Autodesk Fusion 360 part; units mm, degrees
(part 5 of 8)
  spline S792 degree 3 poles (24.0351, 9.5293) (23.3482, 9.5293) (23.0556, 8.9736) (22.8466, 8.9736) knots 0 0 0 0 1 1 1 1
  spline S793 degree 3 poles (22.8466, 8.9736) (22.2105, 8.9736) (21.3624, 9.9262) (21.3624, 10.7728) knots 0 0 0 0 1 1 1 1
  spline S794 degree 3 poles (21.3624, 10.7728) (21.3624, 11.8842) (22.739, 13.0748) (24.3546, 13.0748) knots 0 0 0 0 1 1 1 1
  spline S795 degree 3 poles (24.3546, 13.0748) (26.2837, 13.0748) (27.8455, 11.3814) (27.8455, 9.3176) knots 0 0 0 0 1 1 1 1
  spline S796 degree 3 poles (27.8455, 9.3176) (27.8455, 7.413) (26.8204, 6.2798) (25.0116, 5.8403) knots 0 0 0 0 0.899792 0.899792 0.899792 0.899792
  spline S797 degree 3 poles (25.0116, 5.8403) (24.8102, 5.7914) (24.5991, 5.751) (24.3785, 5.7192) knots 0.899792 0.899792 0.899792 0.899792 1 1 1 1
  spline S798 degree 3 poles (24.3785, 5.7192) (25.0522, 5.3732) (25.6655, 4.9493) (26.2098, 4.4555) knots 0 0 0 0 0.233548 0.233548 0.233548 0.233548
  ellipse E21 centre (19.5885, -1.7408) end of major axis (19.5885, -11.5568) minor radius 8.5372 (19.5885, -11.5568) -> (26.2098, 4.4555) ccw
  spline S799 degree 3 poles (19.5885, -11.5568) (19.4017, -11.5543) (19.2169, -11.5473) (19.0342, -11.5361) knots 0.009853 0.009853 0.009853 0.009853 0.044162 0.044162 0.044162 0.044162
  spline S800 degree 3 poles (207.0718, -10.6848) (207.0718, -10.1028) (207.4951, -6.9807) (207.4951, -6.769) knots 0 0 0 0 1 1 1 1
  spline S801 degree 3 poles (207.4951, -6.769) (207.4951, -6.9807) (207.0718, -10.1028) (207.0718, -10.6848) knots -1 -1 -1 -1 0 0 0 0
  spline S802 degree 3 poles (9.0107, -11.2935) (7.9525, -11.2406) (6.6827, -11.2142) (5.5155, -11.2142) knots 0 0 0 0 1 1 1 1
  spline S803 degree 3 poles (5.5155, -11.2142) (6.6827, -11.2142) (7.9525, -11.2406) (9.0107, -11.2935) knots -1 -1 -1 -1 0 0 0 0
  spline S804 degree 3 poles (-20.2282, 3.0734) (-20.1993, 0.0308) (-10.7804, 0.4806) (-10.7804, -6.1341) knots 0 0 0 0 1 1 1 1
  spline S805 degree 3 poles (-10.7804, -6.1341) (-10.7804, 0.4806) (-20.1993, 0.0308) (-20.2282, 3.0734) knots -1 -1 -1 -1 0 0 0 0
  spline S806 degree 3 poles (25.2803, 8.4181) (25.2803, 9.0001) (24.9608, 9.5293) (24.0351, 9.5293) knots 0 0 0 0 1 1 1 1
  spline S807 degree 3 poles (24.0351, 9.5293) (24.9608, 9.5293) (25.2803, 9.0001) (25.2803, 8.4181) knots -1 -1 -1 -1 0 0 0 0
  spline S808 degree 3 poles (312.7442, 4.1318) (313.1411, 5.2166) (311.4213, 5.1902) (311.4213, 5.587) knots 0 0 0 0 1 1 1 1
  spline S809 degree 3 poles (311.4213, 5.587) (311.4213, 5.1902) (313.1411, 5.2166) (312.7442, 4.1318) knots -1 -1 -1 -1 0 0 0 0
  spline S810 degree 3 poles (-61.1571, -0.6308) (-61.1571, 4.158) (-58.5644, 6.7775) (-53.9628, 6.7775) knots 0 0 0 0 0.999995 0.999995 0.999995 0.999995
  spline S811 degree 3 poles (-53.9628, 6.7775) (-58.5644, 6.7775) (-61.1571, 4.158) (-61.1571, -0.6308) knots -0.999995 -0.999995 -0.999995 -0.999995 0 0 0 0
  line L198 (311.1567, -0.3132) -> (306.2614, -0.2867)
  line L199 (306.2614, -0.2867) -> (308.7223, -7.2188)
  line L200 (308.7223, -7.2188) -> (311.1567, -0.3132)
  line L201 (305.6267, 1.5654) -> (311.8446, 1.6183)
  line L202 (311.8446, 1.6183) -> (312.7442, 4.1318)
  spline S812 degree 3 poles (312.7442, 4.1318) (313.1411, 5.2166) (311.4213, 5.1902) (311.4213, 5.587) knots 0 0 0 0 1 1 1 1
  spline S813 degree 3 poles (311.4213, 5.587) (311.4213, 5.9045) (311.7123, 6.5131) (311.924, 6.4866) knots 0 0 0 0 1 1 1 1
  spline S814 degree 3 poles (311.924, 6.4866) (312.3209, 6.4337) (313.1149, 6.4072) (313.9086, 6.4072) knots 0 0 0 0 1 1 1 1
  spline S815 degree 3 poles (313.9086, 6.4072) (314.7024, 6.4072) (315.4961, 6.4337) (315.893, 6.4866) knots 0 0 0 0 1 1 1 1
  spline S816 degree 3 poles (315.893, 6.4866) (316.1311, 6.5131) (316.3957, 5.9045) (316.3957, 5.587) knots 0 0 0 0 1 1 1 1
  spline S817 degree 3 poles (316.3957, 5.587) (316.3957, 5.1902) (315.2051, 5.1902) (314.8347, 4.1318) knots 0 0 0 0 1 1 1 1
  line L203 (314.8347, 4.1318) -> (309.9129, -9.6794)
  spline S818 degree 3 poles (309.9129, -9.6794) (310.3627, -10.0234) (310.8919, -10.1557) (310.8919, -10.4203) knots 0 0 0 0 1 1 1 1
  spline S819 degree 3 poles (310.8919, -10.4203) (310.8919, -10.7378) (310.6011, -11.3225) (310.3894, -11.2934) knots 0 0 0 0 1 1 1 1
  spline S820 degree 3 poles (310.3894, -11.2934) (308.5106, -11.1346) (306.4998, -11.2934) (305.5999, -11.2934) knots 0 0 0 0 1 1 1 1
  spline S821 degree 3 poles (305.5999, -11.2934) (304.7003, -11.2934) (304.4358, -11.1346) (304.277, -10.6848) knots 0 0 0 0 1 1 1 1
  line L204 (304.277, -10.6848) -> (299.0115, 4.1318)
  spline S822 degree 3 poles (299.0115, 4.1318) (298.6411, 5.2166) (297.4505, 5.1902) (297.4505, 5.587) knots 0 0 0 0 1 1 1 1
  spline S823 degree 3 poles (297.4505, 5.587) (297.4505, 5.9045) (297.7151, 6.4866) (297.9265, 6.4866) knots 0 0 0 0 1 1 1 1
  spline S824 degree 3 poles (297.9265, 6.4866) (298.9851, 6.4337) (300.3609, 6.4072) (301.737, 6.4072) knots 0 0 0 0 1 1 1 1
  spline S825 degree 3 poles (301.737, 6.4072) (303.1129, 6.4072) (304.4622, 6.4337) (305.5206, 6.4866) knots 0 0 0 0 1 1 1 1
  spline S826 degree 3 poles (305.5206, 6.4866) (305.7322, 6.4866) (306.0235, 5.9045) (306.0235, 5.587) knots 0 0 0 0 1 1 1 1
  spline S827 degree 3 poles (306.0235, 5.587) (306.0235, 5.1902) (304.3299, 5.2166) (304.7004, 4.1318) knots 0 0 0 0 1 1 1 1
  line L205 (304.7004, 4.1318) -> (305.6267, 1.5654)
  line L206 (-32.4486, -8.7797) -> (-32.4486, 4.1582)
  line L207 (-32.4486, 4.1582) -> (-32.4486, -8.7797)
  spline S828 degree 3 poles (27.8455, 9.3176) (27.8455, 7.413) (26.8204, 6.2798) (25.0116, 5.8403) knots 0 0 0 0 0.899792 0.899792 0.899792 0.899792
  spline S829 degree 3 poles (25.0116, 5.8403) (26.8204, 6.2798) (27.8455, 7.413) (27.8455, 9.3176) knots -0.899792 -0.899792 -0.899792 -0.899792 0 0 0 0
  line L208 (182.2539, -3.885) -> (182.2539, -8.965)
  line L209 (182.2539, -8.965) -> (182.2539, -3.885)
  spline S830 degree 3 poles (180.7986, -10.4203) (180.7986, -10.0234) (182.2539, -10.1028) (182.2539, -8.965) knots 0 0 0 0 1 1 1 1
  line L210 (182.2539, -8.965) -> (182.2539, -3.885)
  line L211 (182.2539, -3.885) -> (175.9039, -3.885)
  line L212 (175.9039, -3.885) -> (175.9039, -8.965)
  spline S831 degree 3 poles (175.9039, -8.965) (175.9039, -10.0763) (177.3326, -9.9969) (177.3326, -10.4203) knots 0 0 0 0 1 1 1 1
  spline S832 degree 3 poles (177.3326, -10.4203) (177.3326, -10.7378) (177.068, -11.3225) (176.8564, -11.2934) knots 0 0 0 0 1 1 1 1
  spline S833 degree 3 poles (176.8564, -11.2934) (175.798, -11.2405) (174.5016, -11.214) (173.2316, -11.214) knots 0 0 0 0 1 1 1 1
  spline S834 degree 3 poles (173.2316, -11.214) (171.9351, -11.214) (170.6386, -11.2405) (169.6068, -11.2934) knots 0 0 0 0 1 1 1 1
  spline S835 degree 3 poles (169.6068, -11.2934) (169.3951, -11.3225) (169.1041, -10.7378) (169.1041, -10.4203) knots 0 0 0 0 1 1 1 1
  spline S836 degree 3 poles (169.1041, -10.4203) (169.1041, -9.9969) (170.5593, -10.0763) (170.5593, -8.965) knots 0 0 0 0 1 1 1 1
  line L213 (170.5593, -8.965) -> (170.5593, 4.1583)
  spline S837 degree 3 poles (170.5593, 4.1583) (170.5593, 5.296) (169.1041, 5.2166) (169.1041, 5.64) knots 0 0 0 0 1 1 1 1
  spline S838 degree 3 poles (169.1041, 5.64) (169.1041, 5.9575) (169.3951, 6.5131) (169.6068, 6.5131) knots 0 0 0 0 1 1 1 1
  spline S839 degree 3 poles (169.6068, 6.5131) (170.6386, 6.4602) (171.9351, 6.4337) (173.2316, 6.4337) knots 0 0 0 0 1 1 1 1
  spline S840 degree 3 poles (173.2316, 6.4337) (174.5016, 6.4337) (175.798, 6.4602) (176.8564, 6.5131) knots 0 0 0 0 1 1 1 1
  spline S841 degree 3 poles (176.8564, 6.5131) (177.068, 6.5131) (177.3326, 5.9575) (177.3326, 5.64) knots 0 0 0 0 1 1 1 1
  spline S842 degree 3 poles (177.3326, 5.64) (177.3326, 5.2166) (175.9039, 5.296) (175.9039, 4.1583) knots 0 0 0 0 1 1 1 1
  line L214 (175.9039, 4.1583) -> (175.9039, -1.9007)
  line L215 (175.9039, -1.9007) -> (182.2539, -1.9007)
  line L216 (182.2539, -1.9007) -> (182.2539, 4.1583)
  spline S843 degree 3 poles (182.2539, 4.1583) (182.2539, 5.296) (180.7986, 5.2166) (180.7986, 5.64) knots 0 0 0 0 1 1 1 1
  spline S844 degree 3 poles (180.7986, 5.64) (180.7986, 5.9575) (181.0897, 6.5131) (181.3014, 6.5131) knots 0 0 0 0 1 1 1 1
  spline S845 degree 3 poles (181.3014, 6.5131) (182.3332, 6.4602) (183.6297, 6.4337) (184.8997, 6.4337) knots 0 0 0 0 1 1 1 1
  spline S846 degree 3 poles (184.8997, 6.4337) (186.1961, 6.4337) (187.4661, 6.4602) (188.5245, 6.5131) knots 0 0 0 0 1 1 1 1
  spline S847 degree 3 poles (188.5245, 6.5131) (188.7626, 6.5131) (189.0272, 5.9575) (189.0272, 5.64) knots 0 0 0 0 1 1 1 1
  spline S848 degree 3 poles (189.0272, 5.64) (189.0272, 5.2166) (187.5984, 5.296) (187.5984, 4.1583) knots 0 0 0 0 1 1 1 1
  line L217 (187.5984, 4.1583) -> (187.5984, -8.965)
  spline S849 degree 3 poles (187.5984, -8.965) (187.5984, -10.0763) (189.0272, -9.9969) (189.0272, -10.4203) knots 0 0 0 0 1 1 1 1
  spline S850 degree 3 poles (189.0272, -10.4203) (189.0272, -10.7378) (188.7626, -11.3225) (188.5245, -11.2934) knots 0 0 0 0 1 1 1 1
  spline S851 degree 3 poles (188.5245, -11.2934) (187.4661, -11.2405) (186.1961, -11.214) (184.8997, -11.214) knots 0 0 0 0 1 1 1 1
  spline S852 degree 3 poles (184.8997, -11.214) (183.6297, -11.214) (182.3332, -11.2405) (181.3014, -11.2934) knots 0 0 0 0 1 1 1 1
  spline S853 degree 3 poles (181.3014, -11.2934) (181.0897, -11.3225) (180.7986, -10.7378) (180.7986, -10.4203) knots 0 0 0 0 1 1 1 1
  spline S854 degree 3 poles (-62.1118, -11.2935) (-62.3212, -11.3227) (-62.5342, -10.7379) (-62.5342, -10.4202) knots 0 0 0 0 1 1 1 1
  spline S855 degree 3 poles (-62.5342, -10.4202) (-62.5342, -10.7379) (-62.3212, -11.3227) (-62.1118, -11.2935) knots -1 -1 -1 -1 0 0 0 0
  spline S856 degree 3 poles (-8.269, 4.1319) (-8.851, 5.1107) (-10.096, 5.2165) (-10.096, 5.6134) knots 0 0 0 0 1 1 1 1
  spline S857 degree 3 poles (-10.096, 5.6134) (-10.096, 5.2165) (-8.851, 5.1107) (-8.269, 4.1319) knots -1 -1 -1 -1 0 0 0 0
  spline S858 degree 3 poles (25.0116, 5.8403) (24.8102, 5.7914) (24.5991, 5.751) (24.3785, 5.7192) knots 0.899792 0.899792 0.899792 0.899792 1 1 1 1
  spline S859 degree 3 poles (24.3785, 5.7192) (24.5991, 5.751) (24.8102, 5.7914) (25.0116, 5.8403) knots -1 -1 -1 -1 -0.899792 -0.899792 -0.899792 -0.899792
  spline S860 degree 3 poles (112.6975, 5.6135) (112.6975, 5.2166) (111.5334, 5.296) (111.3746, 4.1583) knots 0 0 0 0 1 1 1 1
  spline S861 degree 3 poles (111.3746, 4.1583) (111.5334, 5.296) (112.6975, 5.2166) (112.6975, 5.6135) knots -1 -1 -1 -1 0 0 0 0
  spline S862 degree 3 poles (208.3682, -6.2663) (208.8709, -6.2663) (208.9503, -9.3619) (213.7393, -9.3619) knots 0 0 0 0 1 1 1 1
  spline S863 degree 3 poles (213.7393, -9.3619) (208.9503, -9.3619) (208.8709, -6.2663) (208.3682, -6.2663) knots -1 -1 -1 -1 0 0 0 0
  spline S864 degree 3 poles (16.2828, -2.3771) (16.2828, 2.518) (17.3668, 4.9254) (19.7498, 4.9254) knots -1 -1 -1 -1 0 0 0 0
  spline S865 degree 3 poles (19.7498, 4.9254) (22.1298, 4.9254) (23.2168, 2.518) (23.2168, -2.3771) knots -1 -1 -1 -1 0 0 0 0
  spline S866 degree 3 poles (23.2168, -2.3771) (23.2168, -7.2718) (22.1298, -9.7058) (19.7498, -9.7058) knots -1 -1 -1 -1 0 0 0 0
  spline S867 degree 3 poles (19.7498, -9.7058) (17.3937, -9.7058) (16.2828, -7.3512) (16.2828, -2.3771) knots -1 -1 -1 -1 0 0 0 0
  ellipse E22 centre (19.5885, -1.7408) end of major axis (19.5885, -11.5568) minor radius 8.5372 (12.3354, 3.4367) -> (19.0342, -11.5361) ccw
  spline S868 degree 3 poles (19.0342, -11.5361) (19.2169, -11.5473) (19.4017, -11.5543) (19.5885, -11.5568) knots -0.044162 -0.044162 -0.044162 -0.044162 -0.009853 -0.009853 -0.009853 -0.009853
  ellipse E23 centre (19.5885, -1.7408) end of major axis (19.5885, -11.5568) minor radius 8.5372 (19.5885, -11.5568) -> (26.2098, 4.4555) ccw
  spline S869 degree 3 poles (26.2098, 4.4555) (25.6655, 4.9493) (25.0522, 5.3732) (24.3785, 5.7192) knots -0.233548 -0.233548 -0.233548 -0.233548 0 0 0 0
  spline S870 degree 3 poles (24.3785, 5.7192) (24.5991, 5.751) (24.8102, 5.7914) (25.0116, 5.8403) knots -1 -1 -1 -1 -0.899792 -0.899792 -0.899792 -0.899792
  spline S871 degree 3 poles (25.0116, 5.8403) (26.8204, 6.2798) (27.8455, 7.413) (27.8455, 9.3176) knots -0.899792 -0.899792 -0.899792 -0.899792 0 0 0 0
  spline S872 degree 3 poles (27.8455, 9.3176) (27.8455, 11.3814) (26.2837, 13.0748) (24.3546, 13.0748) knots -1 -1 -1 -1 0 0 0 0
  spline S873 degree 3 poles (24.3546, 13.0748) (22.739, 13.0748) (21.3624, 11.8842) (21.3624, 10.7728) knots -1 -1 -1 -1 0 0 0 0
  spline S874 degree 3 poles (21.3624, 10.7728) (21.3624, 9.9262) (22.2105, 8.9736) (22.8466, 8.9736) knots -1 -1 -1 -1 0 0 0 0
  spline S875 degree 3 poles (22.8466, 8.9736) (23.0556, 8.9736) (23.3482, 9.5293) (24.0351, 9.5293) knots -1 -1 -1 -1 0 0 0 0
  spline S876 degree 3 poles (24.0351, 9.5293) (24.9608, 9.5293) (25.2803, 9.0001) (25.2803, 8.4181) knots -1 -1 -1 -1 0 0 0 0
  spline S877 degree 3 poles (25.2803, 8.4181) (25.2803, 7.8624) (24.8832, 7.307) (24.1426, 7.307) knots -1 -1 -1 -1 0 0 0 0
  spline S878 degree 3 poles (24.1426, 7.307) (22.2105, 7.307) (19.1944, 12.0165) (15.2526, 12.1222) knots -1 -1 -1 -1 0 0 0 0
  spline S879 degree 3 poles (15.2526, 12.1222) (12.9234, 12.1751) (11.3616, 10.4553) (11.3616, 8.4444) knots -1 -1 -1 -1 0 0 0 0
  spline S880 degree 3 poles (11.3616, 8.4444) (11.3616, 6.6189) (12.7113, 6.1955) (13.3205, 6.1955) knots -1 -1 -1 -1 0 0 0 0
  spline S881 degree 3 poles (13.3205, 6.1955) (13.5056, 6.1955) (13.637, 6.2221) (13.637, 6.2749) knots -1 -1 -1 -1 0 0 0 0
  spline S882 degree 3 poles (13.637, 6.2749) (13.637, 6.8569) (13.9565, 7.2804) (14.9092, 7.2804) knots -1 -1 -1 -1 0 0 0 0
  spline S883 degree 3 poles (14.9092, 7.2804) (15.2092, 7.2804) (15.5699, 7.2326) (15.9755, 7.1529) knots -1 -1 -1 -1 -0.594925 -0.594925 -0.594925 -0.594925
  spline S884 degree 3 poles (15.9755, 7.1529) (16.5713, 7.0359) (17.2638, 6.85) (18.0029, 6.6455) knots -0.594925 -0.594925 -0.594925 -0.594925 0 0 0 0
  spline S885 degree 3 poles (18.0029, 6.6455) (15.615, 6.2706) (13.6571, 5.1309) (12.3354, 3.4367) knots -1 -1 -1 -1 -0.475314 -0.475314 -0.475314 -0.475314
  spline S886 degree 3 poles (-31.4184, -9.3619) (-28.3745, -9.3619) (-27.1051, -5.7372) (-26.6033, -5.7372) knots 0 0 0 0 1 1 1 1
  spline S887 degree 3 poles (-26.6033, -5.7372) (-27.1051, -5.7372) (-28.3745, -9.3619) (-31.4184, -9.3619) knots -1 -1 -1 -1 0 0 0 0
  spline S888 degree 3 poles (-125.7439, 6.5132) (-125.5308, 6.5132) (-125.2401, 5.9575) (-125.2401, 5.64) knots 0 0 0 0 1 1 1 1
  spline S889 degree 3 poles (-125.2401, 5.64) (-125.2401, 5.9575) (-125.5308, 6.5132) (-125.7439, 6.5132) knots -1 -1 -1 -1 0 0 0 0
  spline S890 degree 3 poles (88.0913, 5.6135) (88.0913, 5.931) (88.3559, 6.5395) (88.5675, 6.5131) knots 0 0 0 0 1 1 1 1
  spline S891 degree 3 poles (88.5675, 6.5131) (88.3559, 6.5395) (88.0913, 5.931) (88.0913, 5.6135) knots -1 -1 -1 -1 0 0 0 0
  line L218 (108.2261, -4.7317) -> (104.2573, 6.5131)
  line L219 (104.2573, 6.5131) -> (108.2261, -4.7317)
  spline S892 degree 3 poles (-161.2467, -8.7798) (-161.4305, -9.1238) (-160.9281, -9.362) (-159.8169, -9.362) knots 0 0 0 0 1 1 1 1
  spline S893 degree 3 poles (-159.8169, -9.362) (-160.9281, -9.362) (-161.4305, -9.1238) (-161.2467, -8.7798) knots -1 -1 -1 -1 0 0 0 0
  spline S894 degree 3 poles (115.1052, 6.5131) (116.9573, 6.4602) (119.2063, 6.4337) (121.4552, 6.4337) knots 0 0 0 0 1 1 1 1
  spline S895 degree 3 poles (121.4552, 6.4337) (119.2063, 6.4337) (116.9573, 6.4602) (115.1052, 6.5131) knots -1 -1 -1 -1 0 0 0 0
  spline S896 degree 3 poles (-153.7301, -10.5524) (-153.8118, -11.1611) (-154.1018, -11.3224) (-154.6329, -11.2934) knots 0 0 0 0 1 1 1 1
  spline S897 degree 3 poles (-154.6329, -11.2934) (-154.1018, -11.3224) (-153.8118, -11.1611) (-153.7301, -10.5524) knots -1 -1 -1 -1 0 0 0 0
  spline S898 degree 3 poles (-154.6329, -11.2934) (-154.1018, -11.3224) (-153.8118, -11.1611) (-153.7301, -10.5524) knots -1 -1 -1 -1 0 0 0 0
  spline S899 degree 3 poles (-153.7301, -10.5524) (-153.6525, -10.1292) (-153.0438, -6.8484) (-153.0438, -6.6368) knots -1 -1 -1 -1 0 0 0 0
  spline S900 degree 3 poles (-153.0438, -6.6368) (-153.0438, -6.4252) (-153.5994, -6.1339) (-153.918, -6.1339) knots -1 -1 -1 -1 0 0 0 0
  spline S901 degree 3 poles (-153.918, -6.1339) (-154.4205, -6.1339) (-155.8503, -9.362) (-159.8169, -9.362) knots -1 -1 -1 -1 0 0 0 0
  spline S902 degree 3 poles (-159.8169, -9.362) (-160.9281, -9.362) (-161.4305, -9.1238) (-161.2467, -8.7798) knots -1 -1 -1 -1 0 0 0 0
  line L220 (-161.2467, -8.7798) -> (-153.4155, 4.1847)
  spline S903 degree 3 poles (-153.4155, 4.1847) (-152.8314, 5.1373) (-152.7783, 5.2166) (-152.7783, 5.6398) knots -1 -1 -1 -1 0 0 0 0
  spline S904 degree 3 poles (-152.7783, 5.6398) (-152.7783, 5.9576) (-153.0438, 6.5132) (-153.2807, 6.5132) knots -1 -1 -1 -1 0 0 0 0
  spline S905 degree 3 poles (-153.2807, 6.5132) (-155.1354, 6.4601) (-157.6232, 6.4339) (-160.1069, 6.4339) knots -1 -1 -1 -1 0 0 0 0
  spline S906 degree 3 poles (-160.1069, 6.4339) (-162.5703, 6.4339) (-165.0581, 6.4601) (-166.9127, 6.5132) knots -1 -1 -1 -1 0 0 0 0
  spline S907 degree 3 poles (-166.9127, 6.5132) (-167.4397, 6.5397) (-167.6766, 6.3543) (-167.8359, 5.746) knots -1 -1 -1 -1 0 0 0 0
  spline S908 degree 3 poles (-167.8359, 5.746) (-167.9421, 5.3489) (-168.657, 2.174) (-168.657, 1.9624) knots -1 -1 -1 -1 0 0 0 0
  spline S909 degree 3 poles (-168.657, 1.9624) (-168.657, 1.7508) (-168.1014, 1.486) (-167.7828, 1.486) knots -1 -1 -1 -1 0 0 0 0
  spline S910 degree 3 poles (-167.7828, 1.486) (-167.2803, 1.486) (-166.2223, 4.5552) (-161.5939, 4.5552) knots -1 -1 -1 -1 0 0 0 0
  spline S911 degree 3 poles (-161.5939, 4.5552) (-160.2417, 4.5552) (-159.6044, 4.2905) (-159.9516, 3.7083) knots -1 -1 -1 -1 0 0 0 0
  line L221 (-159.9516, 3.7083) -> (-167.599, -8.9649)
  spline S912 degree 3 poles (-167.599, -8.9649) (-168.1791, -9.9175) (-168.126, -10.0234) (-168.126, -10.42) knots -1 -1 -1 -1 0 0 0 0
  spline S913 degree 3 poles (-168.126, -10.42) (-168.126, -10.7378) (-167.8359, -11.3224) (-167.6235, -11.2934) knots -1 -1 -1 -1 0 0 0 0
  spline S914 degree 3 poles (-167.6235, -11.2934) (-163.9224, -11.1901) (-158.334, -11.2138) (-154.6329, -11.2934) knots -1 -1 -1 -1 0 0 0 0
  spline S915 degree 3 poles (-99.0459, -5.0229) (-97.7765, -0.8688) (-95.2114, 3.9993) (-94.7607, 6.5129) knots 0 0 0 0 1 1 1 1
  spline S916 degree 3 poles (-94.7607, 6.5129) (-95.2114, 3.9993) (-97.7765, -0.8688) (-99.0459, -5.0229) knots -1 -1 -1 -1 0 0 0 0
  line L222 (-161.2467, -8.7798) -> (-153.4155, 4.1847)
  line L223 (-153.4155, 4.1847) -> (-161.2467, -8.7798)
  spline S917 degree 3 poles (-167.6235, -11.2934) (-167.8359, -11.3224) (-168.126, -10.7378) (-168.126, -10.42) knots 0 0 0 0 1 1 1 1
  spline S918 degree 3 poles (-168.126, -10.42) (-168.126, -10.7378) (-167.8359, -11.3224) (-167.6235, -11.2934) knots -1 -1 -1 -1 0 0 0 0
  spline S919 degree 3 poles (-84.4965, -8.9388) (-84.1247, -9.9972) (-82.9079, -9.9705) (-82.9079, -10.3938) knots 0 0 0 0 1 1 1 1
  spline S920 degree 3 poles (-82.9079, -10.3938) (-82.9079, -9.9705) (-84.1247, -9.9972) (-84.4965, -8.9388) knots -1 -1 -1 -1 0 0 0 0
  spline S921 degree 3 poles (-153.7301, -10.5524) (-153.8118, -11.1611) (-154.1018, -11.3224) (-154.6329, -11.2934) knots 0 0 0 0 1 1 1 1
  spline S922 degree 3 poles (-154.6329, -11.2934) (-158.334, -11.2138) (-163.9224, -11.1901) (-167.6235, -11.2934) knots 0 0 0 0 1 1 1 1
  spline S923 degree 3 poles (-167.6235, -11.2934) (-167.8359, -11.3224) (-168.126, -10.7378) (-168.126, -10.42) knots 0 0 0 0 1 1 1 1
  spline S924 degree 3 poles (-168.126, -10.42) (-168.126, -10.0234) (-168.1791, -9.9175) (-167.599, -8.9649) knots 0 0 0 0 1 1 1 1
  line L224 (-167.599, -8.9649) -> (-159.9516, 3.7083)
  spline S925 degree 3 poles (-159.9516, 3.7083) (-159.6044, 4.2905) (-160.2417, 4.5552) (-161.5939, 4.5552) knots 0 0 0 0 1 1 1 1
  spline S926 degree 3 poles (-161.5939, 4.5552) (-166.2223, 4.5552) (-167.2803, 1.486) (-167.7828, 1.486) knots 0 0 0 0 1 1 1 1
  spline S927 degree 3 poles (-167.7828, 1.486) (-168.1014, 1.486) (-168.657, 1.7508) (-168.657, 1.9624) knots 0 0 0 0 1 1 1 1
  spline S928 degree 3 poles (-168.657, 1.9624) (-168.657, 2.174) (-167.9421, 5.3489) (-167.8359, 5.746) knots 0 0 0 0 1 1 1 1
  spline S929 degree 3 poles (-167.8359, 5.746) (-167.6766, 6.3543) (-167.4397, 6.5397) (-166.9127, 6.5132) knots 0 0 0 0 1 1 1 1
  spline S930 degree 3 poles (-166.9127, 6.5132) (-165.0581, 6.4601) (-162.5703, 6.4339) (-160.1069, 6.4339) knots 0 0 0 0 1 1 1 1
  spline S931 degree 3 poles (-160.1069, 6.4339) (-157.6232, 6.4339) (-155.1354, 6.4601) (-153.2807, 6.5132) knots 0 0 0 0 1 1 1 1
  spline S932 degree 3 poles (-153.2807, 6.5132) (-153.0438, 6.5132) (-152.7783, 5.9576) (-152.7783, 5.6398) knots 0 0 0 0 1 1 1 1
  spline S933 degree 3 poles (-152.7783, 5.6398) (-152.7783, 5.2166) (-152.8314, 5.1373) (-153.4155, 4.1847) knots 0 0 0 0 1 1 1 1
  line L225 (-153.4155, 4.1847) -> (-161.2467, -8.7798)
  spline S934 degree 3 poles (-161.2467, -8.7798) (-161.4305, -9.1238) (-160.9281, -9.362) (-159.8169, -9.362) knots 0 0 0 0 1 1 1 1
  spline S935 degree 3 poles (-159.8169, -9.362) (-155.8503, -9.362) (-154.4205, -6.1339) (-153.918, -6.1339) knots 0 0 0 0 1 1 1 1
  spline S936 degree 3 poles (-153.918, -6.1339) (-153.5994, -6.1339) (-153.0438, -6.4252) (-153.0438, -6.6368) knots 0 0 0 0 1 1 1 1
  spline S937 degree 3 poles (-153.0438, -6.6368) (-153.0438, -6.8484) (-153.6525, -10.1292) (-153.7301, -10.5524) knots 0 0 0 0 1 1 1 1
  spline S938 degree 3 poles (-104.7093, -10.3938) (-104.7093, -9.9705) (-103.0155, -9.9972) (-103.3873, -8.9122) knots 0 0 0 0 1 1 1 1
  spline S939 degree 3 poles (-103.3873, -8.9122) (-103.0155, -9.9972) (-104.7093, -9.9705) (-104.7093, -10.3938) knots -1 -1 -1 -1 0 0 0 0
  spline S940 degree 3 poles (-119.6048, 4.132) (-118.9691, 5.0843) (-120.4768, 5.2164) (-120.4768, 5.6133) knots 0 0 0 0 1 1 1 1
  spline S941 degree 3 poles (-120.4768, 5.6133) (-120.4768, 5.2164) (-118.9691, 5.0843) (-119.6048, 4.132) knots -1 -1 -1 -1 0 0 0 0
  spline S942 degree 3 poles (58.909, 4.9256) (61.2897, 4.9256) (62.3744, 2.5179) (62.3744, -2.3768) knots -1 -1 -1 -1 0 0 0 0
  spline S943 degree 3 poles (58.909, 4.9256) (61.2897, 4.9256) (62.3744, 2.5179) (62.3744, -2.3768) knots -1 -1 -1 -1 0 0 0 0
  spline S944 degree 3 poles (62.3744, -2.3768) (62.3744, -7.2715) (61.2897, -9.7058) (58.909, -9.7058) knots -1 -1 -1 -1 0 0 0 0
  spline S945 degree 3 poles (62.3744, -2.3768) (62.3744, -7.2715) (61.2897, -9.7058) (58.909, -9.7058) knots -1 -1 -1 -1 0 0 0 0
  spline S946 degree 3 poles (-134.5263, 5.64) (-134.5263, 5.9575) (-134.2356, 6.5132) (-134.0225, 6.5132) knots 0 0 0 0 1 1 1 1
  spline S947 degree 3 poles (-134.0225, 6.5132) (-134.2356, 6.5132) (-134.5263, 5.9575) (-134.5263, 5.64) knots -1 -1 -1 -1 0 0 0 0
  line L226 (126.9057, -8.965) -> (126.9057, 4.1847)
  line L227 (126.9057, 4.1847) -> (126.9057, -8.965)
  spline S948 degree 3 poles (113.3325, 1.9622) (113.3325, 2.1739) (114.0469, 5.3489) (114.1527, 5.7458) knots 0 0 0 0 1 1 1 1
  spline S949 degree 3 poles (114.1527, 5.7458) (114.0469, 5.3489) (113.3325, 2.1739) (113.3325, 1.9622) knots -1 -1 -1 -1 0 0 0 0
  spline S950 degree 3 poles (128.3344, 5.64) (128.3344, 5.2166) (126.9057, 5.296) (126.9057, 4.1847) knots 0 0 0 0 1 1 1 1
  spline S951 degree 3 poles (126.9057, 4.1847) (126.9057, 5.296) (128.3344, 5.2166) (128.3344, 5.64) knots -1 -1 -1 -1 0 0 0 0
  spline S952 degree 3 poles (114.1527, 5.7458) (114.338, 6.3543) (114.5496, 6.5395) (115.1052, 6.5131) knots 0 0 0 0 1 1 1 1
  spline S953 degree 3 poles (115.1052, 6.5131) (114.5496, 6.5395) (114.338, 6.3543) (114.1527, 5.7458) knots -1 -1 -1 -1 0 0 0 0
  spline S954 degree 3 poles (127.8317, 6.5131) (128.0698, 6.5131) (128.3344, 5.9575) (128.3344, 5.64) knots 0 0 0 0 1 1 1 1
  spline S955 degree 3 poles (128.3344, 5.64) (128.3344, 5.9575) (128.0698, 6.5131) (127.8317, 6.5131) knots -1 -1 -1 -1 0 0 0 0
  spline S956 degree 3 poles (126.9057, -8.965) (126.9057, -10.1028) (128.3344, -9.9969) (128.3344, -10.4203) knots 0 0 0 0 1 1 1 1
  spline S957 degree 3 poles (128.3344, -10.4203) (128.3344, -9.9969) (126.9057, -10.1028) (126.9057, -8.965) knots -1 -1 -1 -1 0 0 0 0
  spline S958 degree 3 poles (121.5611, 3.7085) (121.5611, 4.3964) (121.27, 4.5552) (119.6296, 4.5552) knots 0 0 0 0 1 1 1 1
  spline S959 degree 3 poles (119.6296, 4.5552) (121.27, 4.5552) (121.5611, 4.3964) (121.5611, 3.7085) knots -1 -1 -1 -1 0 0 0 0
  spline S960 degree 3 poles (128.3344, -10.4203) (128.3344, -10.7378) (128.0698, -11.3225) (127.8317, -11.2934) knots 0 0 0 0 1 1 1 1
  spline S961 degree 3 poles (127.8317, -11.2934) (128.0698, -11.3225) (128.3344, -10.7378) (128.3344, -10.4203) knots -1 -1 -1 -1 0 0 0 0
  spline S962 degree 3 poles (-124.9494, -11.2934) (-125.1587, -11.3224) (-125.4494, -10.7376) (-125.4494, -10.4202) knots 0 0 0 0 1 1 1 1
  spline S963 degree 3 poles (-125.4494, -10.4202) (-125.4494, -10.7376) (-125.1587, -11.3224) (-124.9494, -11.2934) knots -1 -1 -1 -1 0 0 0 0
  spline S964 degree 3 poles (119.6296, 4.5552) (115.7667, 4.5552) (114.7348, 1.486) (114.2321, 1.486) knots 0 0 0 0 1 1 1 1
  spline S965 degree 3 poles (114.2321, 1.486) (114.7348, 1.486) (115.7667, 4.5552) (119.6296, 4.5552) knots -1 -1 -1 -1 0 0 0 0
  spline S966 degree 3 poles (127.8317, -11.2934) (126.7734, -11.2405) (125.5034, -11.214) (124.2069, -11.214) knots 0 0 0 0 1 1 1 1
  spline S967 degree 3 poles (124.2069, -11.214) (125.5034, -11.214) (126.7734, -11.2405) (127.8317, -11.2934) knots -1 -1 -1 -1 0 0 0 0
  spline S968 degree 3 poles (114.2321, 1.486) (113.9146, 1.486) (113.3325, 1.7506) (113.3325, 1.9622) knots 0 0 0 0 1 1 1 1
  spline S969 degree 3 poles (113.3325, 1.9622) (113.3325, 1.7506) (113.9146, 1.486) (114.2321, 1.486) knots -1 -1 -1 -1 0 0 0 0
  line L228 (-122.9922, -1.0805) -> (-126.4299, 4.1584)
  line L229 (-126.4299, 4.1584) -> (-122.9922, -1.0805)
  line L230 (121.5611, 3.7085) -> (121.5611, -8.965)
  line L231 (121.5611, -8.965) -> (121.5611, 3.7085)
  spline S970 degree 3 poles (-129.8948, 6.4338) (-128.3368, 6.4338) (-126.802, 6.4601) (-125.7439, 6.5132) knots 0 0 0 0 1 1 1 1
  spline S971 degree 3 poles (-125.7439, 6.5132) (-126.802, 6.4601) (-128.3368, 6.4338) (-129.8948, 6.4338) knots -1 -1 -1 -1 0 0 0 0
  spline S972 degree 3 poles (238.9803, 5.64) (238.9803, 5.2166) (237.5515, 5.296) (237.5515, 4.1847) knots 0 0 0 0 1 1 1 1
  spline S973 degree 3 poles (237.5515, 4.1847) (237.5515, 5.296) (238.9803, 5.2166) (238.9803, 5.64) knots -1 -1 -1 -1 0 0 0 0
  line L232 (232.2072, 3.7085) -> (232.2072, -1.8213)
  line L233 (232.2072, -1.8213) -> (232.2072, 3.7085)
  spline S974 degree 3 poles (238.4778, 6.5131) (238.7157, 6.5131) (238.9803, 5.9575) (238.9803, 5.64) knots 0 0 0 0 1 1 1 1
  spline S975 degree 3 poles (238.9803, 5.64) (238.9803, 5.9575) (238.7157, 6.5131) (238.4778, 6.5131) knots -1 -1 -1 -1 0 0 0 0
  spline S976 degree 3 poles (232.2072, 3.7085) (232.2072, 4.3964) (231.9161, 4.5816) (230.2757, 4.5816) knots 0 0 0 0 1 1 1 1
  spline S977 degree 3 poles (230.2757, 4.5816) (231.9161, 4.5816) (232.2072, 4.3964) (232.2072, 3.7085) knots -1 -1 -1 -1 0 0 0 0
  spline S978 degree 3 poles (231.7839, 6.4337) (234.1913, 6.4337) (236.6255, 6.4602) (238.4778, 6.5131) knots 0 0 0 0 1 1 1 1
  spline S979 degree 3 poles (238.4778, 6.5131) (236.6255, 6.4602) (234.1913, 6.4337) (231.7839, 6.4337) knots -1 -1 -1 -1 0 0 0 0
  spline S980 degree 3 poles (230.2757, 4.5816) (225.4868, 4.5816) (224.7195, 1.486) (224.2168, 1.486) knots 0 0 0 0 1 1 1 1
  spline S981 degree 3 poles (224.2168, 1.486) (224.7195, 1.486) (225.4868, 4.5816) (230.2757, 4.5816) knots -1 -1 -1 -1 0 0 0 0
  spline S982 degree 3 poles (225.0899, 6.5131) (226.942, 6.4602) (229.3497, 6.4337) (231.7839, 6.4337) knots 0 0 0 0 1 1 1 1
  spline S983 degree 3 poles (231.7839, 6.4337) (229.3497, 6.4337) (226.942, 6.4602) (225.0899, 6.5131) knots -1 -1 -1 -1 0 0 0 0
  spline S984 degree 3 poles (224.2168, 1.486) (223.8993, 1.486) (223.3172, 1.7506) (223.3172, 1.9622) knots 0 0 0 0 1 1 1 1
  spline S985 degree 3 poles (223.3172, 1.9622) (223.3172, 1.7506) (223.8993, 1.486) (224.2168, 1.486) knots -1 -1 -1 -1 0 0 0 0
  spline S986 degree 3 poles (224.1374, 5.7458) (224.3226, 6.3543) (224.5343, 6.5395) (225.0899, 6.5131) knots 0 0 0 0 1 1 1 1
  spline S987 degree 3 poles (225.0899, 6.5131) (224.5343, 6.5395) (224.3226, 6.3543) (224.1374, 5.7458) knots -1 -1 -1 -1 0 0 0 0
  spline S988 degree 3 poles (224.9047, -6.2663) (225.4074, -6.2663) (225.4868, -9.3619) (230.2757, -9.3619) knots 0 0 0 0 1 1 1 1
  spline S989 degree 3 poles (230.2757, -9.3619) (225.4868, -9.3619) (225.4074, -6.2663) (224.9047, -6.2663) knots -1 -1 -1 -1 0 0 0 0
  spline S990 degree 3 poles (267.4219, -11.558) (265.305, -11.558) (264.326, -11.0288) (263.4264, -11.0288) knots 0 0 0 0 1 1 1 1
  spline S991 degree 3 poles (263.4264, -11.0288) (264.326, -11.0288) (265.305, -11.558) (267.4219, -11.558) knots -1 -1 -1 -1 0 0 0 0
  spline S992 degree 3 poles (261.6537, -5.7371) (262.1297, -5.7371) (263.4529, -9.653) (266.6546, -9.653) knots 0 0 0 0 1 1 1 1
  spline S993 degree 3 poles (266.6546, -9.653) (263.4529, -9.653) (262.1297, -5.7371) (261.6537, -5.7371) knots -1 -1 -1 -1 0 0 0 0
  spline S994 degree 3 poles (224.0316, -6.769) (224.0316, -6.5573) (224.5872, -6.2663) (224.9047, -6.2663) knots 0 0 0 0 1 1 1 1
  spline S995 degree 3 poles (224.9047, -6.2663) (224.5872, -6.2663) (224.0316, -6.5573) (224.0316, -6.769) knots -1 -1 -1 -1 0 0 0 0
  line L234 (232.2072, -3.6734) -> (232.2072, -8.7798)
  line L235 (232.2072, -8.7798) -> (232.2072, -3.6734)
  spline S996 degree 3 poles (230.2757, -9.3619) (231.8632, -9.3619) (232.2072, -9.4148) (232.2072, -8.7798) knots 0 0 0 0 1 1 1 1
  line L236 (232.2072, -8.7798) -> (232.2072, -3.6734)
  line L237 (232.2072, -3.6734) -> (230.3551, -3.7263)
  spline S997 degree 3 poles (230.3551, -3.7263) (228.1855, -3.7792) (228.3443, -6.5044) (227.5505, -6.5044) knots 0 0 0 0 1 1 1 1
  spline S998 degree 3 poles (227.5505, -6.5044) (227.233, -6.5044) (226.6509, -6.2134) (226.6509, -6.0017) knots 0 0 0 0 1 1 1 1
  spline S999 degree 3 poles (226.6509, -6.0017) (226.7832, -3.8321) (226.7832, -1.6625) (226.6509, 0.507) knots 0 0 0 0 1 1 1 1
  spline S1000 degree 3 poles (226.6509, 0.507) (226.6509, 0.7187) (227.233, 1.0097) (227.5505, 1.0097) knots 0 0 0 0 1 1 1 1
  spline S1001 degree 3 poles (227.5505, 1.0097) (228.3443, 1.0097) (228.1855, -1.7155) (230.3551, -1.7684) knots 0 0 0 0 1 1 1 1
  line L238 (230.3551, -1.7684) -> (232.2072, -1.8213)
  line L239 (232.2072, -1.8213) -> (232.2072, 3.7085)
  spline S1002 degree 3 poles (232.2072, 3.7085) (232.2072, 4.3964) (231.9161, 4.5816) (230.2757, 4.5816) knots 0 0 0 0 1 1 1 1
  spline S1003 degree 3 poles (230.2757, 4.5816) (225.4868, 4.5816) (224.7195, 1.486) (224.2168, 1.486) knots 0 0 0 0 1 1 1 1
  spline S1004 degree 3 poles (224.2168, 1.486) (223.8993, 1.486) (223.3172, 1.7506) (223.3172, 1.9622) knots 0 0 0 0 1 1 1 1
  spline S1005 degree 3 poles (223.3172, 1.9622) (223.3172, 2.1739) (224.0316, 5.3489) (224.1374, 5.7458) knots 0 0 0 0 1 1 1 1
  spline S1006 degree 3 poles (224.1374, 5.7458) (224.3226, 6.3543) (224.5343, 6.5395) (225.0899, 6.5131) knots 0 0 0 0 1 1 1 1
  spline S1007 degree 3 poles (225.0899, 6.5131) (226.942, 6.4602) (229.3497, 6.4337) (231.7839, 6.4337) knots 0 0 0 0 1 1 1 1
  spline S1008 degree 3 poles (231.7839, 6.4337) (234.1913, 6.4337) (236.6255, 6.4602) (238.4778, 6.5131) knots 0 0 0 0 1 1 1 1
  spline S1009 degree 3 poles (238.4778, 6.5131) (238.7157, 6.5131) (238.9803, 5.9575) (238.9803, 5.64) knots 0 0 0 0 1 1 1 1
  spline S1010 degree 3 poles (238.9803, 5.64) (238.9803, 5.2166) (237.5515, 5.296) (237.5515, 4.1847) knots 0 0 0 0 1 1 1 1
  line L240 (237.5515, 4.1847) -> (237.5515, -8.9386)
  spline S1011 degree 3 poles (237.5515, -8.9386) (237.5515, -10.0763) (238.9803, -9.9969) (238.9803, -10.3938) knots 0 0 0 0 1 1 1 1
  spline S1012 degree 3 poles (238.9803, -10.3938) (238.9803, -10.7113) (238.7157, -11.2934) (238.4778, -11.2934) knots 0 0 0 0 1 1 1 1
  spline S1013 degree 3 poles (238.4778, -11.2934) (236.7313, -11.2405) (234.3236, -11.214) (231.8897, -11.214) knots 0 0 0 0 1 1 1 1
  spline S1014 degree 3 poles (231.8897, -11.214) (229.1645, -11.214) (226.4128, -11.2405) (224.4549, -11.2934) knots 0 0 0 0 1 1 1 1
  spline S1015 degree 3 poles (224.4549, -11.2934) (223.9257, -11.3225) (223.6347, -11.1611) (223.6347, -10.6848) knots 0 0 0 0 1 1 1 1
  spline S1016 degree 3 poles (223.6347, -10.6848) (223.6347, -10.1028) (224.0316, -6.9807) (224.0316, -6.769) knots 0 0 0 0 1 1 1 1
  spline S1017 degree 3 poles (224.0316, -6.769) (224.0316, -6.5573) (224.5872, -6.2663) (224.9047, -6.2663) knots 0 0 0 0 1 1 1 1
  spline S1018 degree 3 poles (224.9047, -6.2663) (225.4074, -6.2663) (225.4868, -9.3619) (230.2757, -9.3619) knots 0 0 0 0 1 1 1 1
  spline S1019 degree 3 poles (230.2757, -9.3619) (231.8632, -9.3619) (232.2072, -9.4148) (232.2072, -8.7798) knots 0 0 0 0 1 1 1 1
  spline S1020 degree 3 poles (232.2072, -8.7798) (232.2072, -9.4148) (231.8632, -9.3619) (230.2757, -9.3619) knots -1 -1 -1 -1 0 0 0 0
  spline S1021 degree 3 poles (232.2072, -8.7798) (232.2072, -9.4148) (231.8632, -9.3619) (230.2757, -9.3619) knots -1 -1 -1 -1 0 0 0 0
  spline S1022 degree 3 poles (230.2757, -9.3619) (225.4868, -9.3619) (225.4074, -6.2663) (224.9047, -6.2663) knots -1 -1 -1 -1 0 0 0 0
  spline S1023 degree 3 poles (224.9047, -6.2663) (224.5872, -6.2663) (224.0316, -6.5573) (224.0316, -6.769) knots -1 -1 -1 -1 0 0 0 0
  spline S1024 degree 3 poles (224.0316, -6.769) (224.0316, -6.9807) (223.6347, -10.1028) (223.6347, -10.6848) knots -1 -1 -1 -1 0 0 0 0
  spline S1025 degree 3 poles (223.6347, -10.6848) (223.6347, -11.1611) (223.9257, -11.3225) (224.4549, -11.2934) knots -1 -1 -1 -1 0 0 0 0
  spline S1026 degree 3 poles (224.4549, -11.2934) (226.4128, -11.2405) (229.1645, -11.214) (231.8897, -11.214) knots -1 -1 -1 -1 0 0 0 0
  spline S1027 degree 3 poles (231.8897, -11.214) (234.3236, -11.214) (236.7313, -11.2405) (238.4778, -11.2934) knots -1 -1 -1 -1 0 0 0 0
  spline S1028 degree 3 poles (238.4778, -11.2934) (238.7157, -11.2934) (238.9803, -10.7113) (238.9803, -10.3938) knots -1 -1 -1 -1 0 0 0 0
  spline S1029 degree 3 poles (238.9803, -10.3938) (238.9803, -9.9969) (237.5515, -10.0763) (237.5515, -8.9386) knots -1 -1 -1 -1 0 0 0 0
  line L241 (237.5515, -8.9386) -> (237.5515, 4.1847)
  spline S1030 degree 3 poles (237.5515, 4.1847) (237.5515, 5.296) (238.9803, 5.2166) (238.9803, 5.64) knots -1 -1 -1 -1 0 0 0 0
  spline S1031 degree 3 poles (238.9803, 5.64) (238.9803, 5.9575) (238.7157, 6.5131) (238.4778, 6.5131) knots -1 -1 -1 -1 0 0 0 0
  spline S1032 degree 3 poles (238.4778, 6.5131) (236.6255, 6.4602) (234.1913, 6.4337) (231.7839, 6.4337) knots -1 -1 -1 -1 0 0 0 0
  spline S1033 degree 3 poles (231.7839, 6.4337) (229.3497, 6.4337) (226.942, 6.4602) (225.0899, 6.5131) knots -1 -1 -1 -1 0 0 0 0
  spline S1034 degree 3 poles (225.0899, 6.5131) (224.5343, 6.5395) (224.3226, 6.3543) (224.1374, 5.7458) knots -1 -1 -1 -1 0 0 0 0
  spline S1035 degree 3 poles (224.1374, 5.7458) (224.0316, 5.3489) (223.3172, 2.1739) (223.3172, 1.9622) knots -1 -1 -1 -1 0 0 0 0
  spline S1036 degree 3 poles (223.3172, 1.9622) (223.3172, 1.7506) (223.8993, 1.486) (224.2168, 1.486) knots -1 -1 -1 -1 0 0 0 0
  spline S1037 degree 3 poles (224.2168, 1.486) (224.7195, 1.486) (225.4868, 4.5816) (230.2757, 4.5816) knots -1 -1 -1 -1 0 0 0 0
  spline S1038 degree 3 poles (230.2757, 4.5816) (231.9161, 4.5816) (232.2072, 4.3964) (232.2072, 3.7085) knots -1 -1 -1 -1 0 0 0 0
  line L242 (232.2072, 3.7085) -> (232.2072, -1.8213)
  line L243 (232.2072, -1.8213) -> (230.3551, -1.7684)
  spline S1039 degree 3 poles (230.3551, -1.7684) (228.1855, -1.7155) (228.3443, 1.0097) (227.5505, 1.0097) knots -1 -1 -1 -1 0 0 0 0
  spline S1040 degree 3 poles (227.5505, 1.0097) (227.233, 1.0097) (226.6509, 0.7187) (226.6509, 0.507) knots -1 -1 -1 -1 0 0 0 0
  spline S1041 degree 3 poles (226.6509, 0.507) (226.7832, -1.6625) (226.7832, -3.8321) (226.6509, -6.0017) knots -1 -1 -1 -1 0 0 0 0
  spline S1042 degree 3 poles (226.6509, -6.0017) (226.6509, -6.2134) (227.233, -6.5044) (227.5505, -6.5044) knots -1 -1 -1 -1 0 0 0 0
  spline S1043 degree 3 poles (227.5505, -6.5044) (228.3443, -6.5044) (228.1855, -3.7792) (230.3551, -3.7263) knots -1 -1 -1 -1 0 0 0 0
  line L244 (230.3551, -3.7263) -> (232.2072, -3.6734)
  line L245 (232.2072, -3.6734) -> (232.2072, -8.7798)
  spline S1044 degree 3 poles (55.4435, -2.3768) (55.4435, 2.5179) (56.5282, 4.9256) (58.909, 4.9256) knots -1 -1 -1 -1 0 0 0 0
  spline S1045 degree 3 poles (55.4435, -2.3768) (55.4435, 2.5179) (56.5282, 4.9256) (58.909, 4.9256) knots -1 -1 -1 -1 0 0 0 0
  spline S1046 degree 3 poles (231.8897, -11.214) (229.1645, -11.214) (226.4128, -11.2405) (224.4549, -11.2934) knots 0 0 0 0 1 1 1 1
  spline S1047 degree 3 poles (224.4549, -11.2934) (226.4128, -11.2405) (229.1645, -11.214) (231.8897, -11.214) knots -1 -1 -1 -1 0 0 0 0
  line L246 (230.3551, -3.7263) -> (232.2072, -3.6734)
  line L247 (232.2072, -3.6734) -> (230.3551, -3.7263)
  spline S1048 degree 3 poles (224.4549, -11.2934) (223.9257, -11.3225) (223.6347, -11.1611) (223.6347, -10.6848) knots 0 0 0 0 1 1 1 1
  spline S1049 degree 3 poles (223.6347, -10.6848) (223.6347, -11.1611) (223.9257, -11.3225) (224.4549, -11.2934) knots -1 -1 -1 -1 0 0 0 0
  spline S1050 degree 3 poles (230.3551, -3.7263) (228.1855, -3.7792) (228.3443, -6.5044) (227.5505, -6.5044) knots 0 0 0 0 1 1 1 1
  spline S1051 degree 3 poles (227.5505, -6.5044) (228.3443, -6.5044) (228.1855, -3.7792) (230.3551, -3.7263) knots -1 -1 -1 -1 0 0 0 0
  spline S1052 degree 3 poles (-132.8326, 4.1584) (-133.4411, 5.1106) (-134.5263, 5.2164) (-134.5263, 5.64) knots 0 0 0 0 1 1 1 1
  spline S1053 degree 3 poles (-134.5263, 5.64) (-134.5263, 5.2164) (-133.4411, 5.1106) (-132.8326, 4.1584) knots -1 -1 -1 -1 0 0 0 0
  spline S1054 degree 3 poles (258.9825, -10.4203) (258.9825, -10.7378) (258.6912, -11.3225) (258.4795, -11.2934) knots 0 0 0 0 1 1 1 1
  spline S1055 degree 3 poles (258.4795, -11.2934) (258.6912, -11.3225) (258.9825, -10.7378) (258.9825, -10.4203) knots -1 -1 -1 -1 0 0 0 0
  spline S1056 degree 3 poles (-161.5939, 4.5552) (-166.2223, 4.5552) (-167.2803, 1.486) (-167.7828, 1.486) knots 0 0 0 0 1 1 1 1
  spline S1057 degree 3 poles (-167.7828, 1.486) (-167.2803, 1.486) (-166.2223, 4.5552) (-161.5939, 4.5552) knots -1 -1 -1 -1 0 0 0 0
  spline S1058 degree 3 poles (157.7825, 12.5985) (159.7669, 12.5985) (161.2221, 12.0958) (161.5661, 11.7518) knots 0 0 0 0 1 1 1 1
  spline S1059 degree 3 poles (161.5661, 11.7518) (161.2221, 12.0958) (159.7669, 12.5985) (157.7825, 12.5985) knots -1 -1 -1 -1 0 0 0 0
  line L248 (70.7082, 2.0681) -> (70.7082, -8.9121)
  spline S1060 degree 3 poles (70.7082, -8.9121) (70.7082, -10.0498) (69.4117, -9.9705) (69.4117, -10.3938) knots -1 -1 -1 -1 0 0 0 0
  spline S1061 degree 3 poles (69.4117, -10.3938) (69.4117, -10.7113) (69.6763, -11.2934) (69.888, -11.2669) knots -1 -1 -1 -1 0 0 0 0
  spline S1062 degree 3 poles (69.888, -11.2669) (70.2848, -11.214) (71.0786, -11.1902) (71.8459, -11.1902) knots -1 -1 -1 -1 0 0 0 0
  spline S1063 degree 3 poles (71.8459, -11.1902) (72.6132, -11.1902) (73.3805, -11.214) (73.7773, -11.2669) knots -1 -1 -1 -1 0 0 0 0
  spline S1064 degree 3 poles (73.7773, -11.2669) (73.989, -11.2934) (74.28, -10.7113) (74.28, -10.3938) knots -1 -1 -1 -1 0 0 0 0
  spline S1065 degree 3 poles (74.28, -10.3938) (74.28, -9.9705) (72.6925, -10.0498) (72.6925, -8.9121) knots -1 -1 -1 -1 0 0 0 0
  line L249 (72.6925, -8.9121) -> (72.6925, 1.486)
  line L250 (72.6925, 1.486) -> (80.3125, -10.6584)
  spline S1066 degree 3 poles (80.3125, -10.6584) (80.5771, -11.0817) (80.7359, -11.2934) (81.6884, -11.2934) knots -1 -1 -1 -1 0 0 0 0
  spline S1067 degree 3 poles (81.6884, -11.2934) (82.5615, -11.2934) (84.8369, -11.1346) (86.7419, -11.2934) knots -1 -1 -1 -1 0 0 0 0
  spline S1068 degree 3 poles (86.7419, -11.2934) (86.9536, -11.3225) (87.2182, -10.6848) (87.2182, -10.3673) knots -1 -1 -1 -1 0 0 0 0
  spline S1069 degree 3 poles (87.2182, -10.3673) (87.2182, -9.9705) (85.9217, -10.0498) (85.9217, -8.9121) knots -1 -1 -1 -1 0 0 0 0
  line L251 (85.9217, -8.9121) -> (85.9217, 4.1583)
  spline S1070 degree 3 poles (85.9217, 4.1583) (85.9217, 5.296) (87.2182, 5.2166) (87.2182, 5.64) knots -1 -1 -1 -1 0 0 0 0
  spline S1071 degree 3 poles (87.2182, 5.64) (87.2182, 5.9575) (86.9536, 6.5395) (86.7419, 6.5131) knots -1 -1 -1 -1 0 0 0 0
  spline S1072 degree 3 poles (86.7419, 6.5131) (86.3186, 6.4602) (85.5513, 6.4337) (84.784, 6.4337) knots -1 -1 -1 -1 0 0 0 0
  spline S1073 degree 3 poles (84.784, 6.4337) (84.0167, 6.4337) (83.2494, 6.4602) (82.8525, 6.5131) knots -1 -1 -1 -1 0 0 0 0
  spline S1074 degree 3 poles (82.8525, 6.5131) (82.6409, 6.5395) (82.3498, 5.931) (82.3498, 5.6135) knots -1 -1 -1 -1 0 0 0 0
  spline S1075 degree 3 poles (82.3498, 5.6135) (82.3498, 5.2166) (83.9373, 5.296) (83.9373, 4.1583) knots -1 -1 -1 -1 0 0 0 0
  line L252 (83.9373, 4.1583) -> (83.9373, -6.2928)
  line L253 (83.9373, -6.2928) -> (76.2909, 5.9045)
  spline S1076 degree 3 poles (76.2909, 5.9045) (76.0263, 6.3014) (75.8675, 6.5131) (74.915, 6.5131) knots -1 -1 -1 -1 0 0 0 0
  spline S1077 degree 3 poles (74.915, 6.5131) (74.0419, 6.5131) (72.6396, 6.3543) (70.7611, 6.5131) knots -1 -1 -1 -1 0 0 0 0
  spline S1078 degree 3 poles (70.7611, 6.5131) (70.5494, 6.5395) (70.1525, 5.931) (70.2584, 5.64) knots -1 -1 -1 -1 0 0 0 0
  spline S1079 degree 3 poles (70.2584, 5.64) (70.5494, 4.8462) (70.7082, 3.7614) (70.7082, 2.0681) knots -1 -1 -1 -1 0 0 0 0
  spline S1080 degree 3 poles (257.527, -8.965) (257.527, -10.0763) (258.9825, -9.9969) (258.9825, -10.4203) knots 0 0 0 0 1 1 1 1
  spline S1081 degree 3 poles (258.9825, -10.4203) (258.9825, -9.9969) (257.527, -10.0763) (257.527, -8.965) knots -1 -1 -1 -1 0 0 0 0
  spline S1082 degree 3 poles (74.28, -10.3938) (74.28, -10.7113) (73.989, -11.2934) (73.7773, -11.2669) knots 0 0 0 0 1 1 1 1
  spline S1083 degree 3 poles (73.7773, -11.2669) (73.989, -11.2934) (74.28, -10.7113) (74.28, -10.3938) knots -1 -1 -1 -1 0 0 0 0
  line L254 (252.1822, 4.026) -> (252.1822, -8.8328)
  line L255 (252.1822, -8.8328) -> (252.1822, 4.026)
  spline S1084 degree 3 poles (70.2584, 5.64) (70.1525, 5.931) (70.5494, 6.5395) (70.7611, 6.5131) knots 0 0 0 0 1 1 1 1
  spline S1085 degree 3 poles (70.7611, 6.5131) (70.5494, 6.5395) (70.1525, 5.931) (70.2584, 5.64) knots -1 -1 -1 -1 0 0 0 0
  spline S1086 degree 3 poles (250.4357, 4.6345) (250.8328, 4.6345) (252.1822, 4.6875) (252.1822, 4.026) knots -1 -1 -1 -1 0 0 0 0
  spline S1087 degree 3 poles (250.4357, 4.6345) (250.8328, 4.6345) (252.1822, 4.6875) (252.1822, 4.026) knots -1 -1 -1 -1 0 0 0 0
  spline S1088 degree 3 poles (-87.2194, -11.1903) (-88.5939, -11.1903) (-89.9722, -11.214) (-91.0313, -11.267) knots 0 0 0 0 1 1 1 1
  spline S1089 degree 3 poles (-91.0313, -11.267) (-89.9722, -11.214) (-88.5939, -11.1903) (-87.2194, -11.1903) knots -1 -1 -1 -1 0 0 0 0
  spline S1090 degree 3 poles (73.7773, -11.2669) (73.3805, -11.214) (72.6132, -11.1902) (71.8459, -11.1902) knots 0 0 0 0 1 1 1 1
  spline S1091 degree 3 poles (71.8459, -11.1902) (72.6132, -11.1902) (73.3805, -11.214) (73.7773, -11.2669) knots -1 -1 -1 -1 0 0 0 0
  spline S1092 degree 3 poles (258.4795, -11.2934) (257.4212, -11.2405) (256.1512, -11.214) (254.9606, -11.214) knots 0 0 0 0 1 1 1 1
  spline S1093 degree 3 poles (254.9606, -11.214) (256.1512, -11.214) (257.4212, -11.2405) (258.4795, -11.2934) knots -1 -1 -1 -1 0 0 0 0
  spline S1094 degree 3 poles (70.7611, 6.5131) (72.6396, 6.3543) (74.0419, 6.5131) (74.915, 6.5131) knots 0 0 0 0 1 1 1 1
  spline S1095 degree 3 poles (74.915, 6.5131) (74.0419, 6.5131) (72.6396, 6.3543) (70.7611, 6.5131) knots -1 -1 -1 -1 0 0 0 0
  spline S1096 degree 3 poles (245.779, -2.4034) (245.779, 2.2797) (247.4194, 4.6345) (250.4357, 4.6345) knots -1 -1 -1 -1 0 0 0 0
  spline S1097 degree 3 poles (245.779, -2.4034) (245.779, 2.2797) (247.4194, 4.6345) (250.4357, 4.6345) knots -1 -1 -1 -1 0 0 0 0
  line L256 (-107.9354, 6.5129) -> (-113.3886, -8.9388)
  line L257 (-113.3886, -8.9388) -> (-107.9354, 6.5129)
  spline S1098 degree 3 poles (71.8459, -11.1902) (71.0786, -11.1902) (70.2848, -11.214) (69.888, -11.2669) knots 0 0 0 0 1 1 1 1
  spline S1099 degree 3 poles (69.888, -11.2669) (70.2848, -11.214) (71.0786, -11.1902) (71.8459, -11.1902) knots -1 -1 -1 -1 0 0 0 0
  spline S1100 degree 3 poles (249.245, 6.5131) (252.0234, 6.4866) (253.1082, 6.4337) (254.9606, 6.4337) knots 0 0 0 0 1 1 1 1
  spline S1101 degree 3 poles (254.9606, 6.4337) (253.1082, 6.4337) (252.0234, 6.4866) (249.245, 6.5131) knots -1 -1 -1 -1 0 0 0 0
  spline S1102 degree 3 poles (74.915, 6.5131) (75.8675, 6.5131) (76.0263, 6.3014) (76.2909, 5.9045) knots 0 0 0 0 1 1 1 1
  spline S1103 degree 3 poles (76.2909, 5.9045) (76.0263, 6.3014) (75.8675, 6.5131) (74.915, 6.5131) knots -1 -1 -1 -1 0 0 0 0
  spline S1104 degree 3 poles (-91.0313, -11.267) (-91.2416, -11.267) (-91.5045, -10.7115) (-91.5045, -10.3938) knots 0 0 0 0 1 1 1 1
  spline S1105 degree 3 poles (-91.5045, -10.3938) (-91.5045, -10.7115) (-91.2416, -11.267) (-91.0313, -11.267) knots -1 -1 -1 -1 0 0 0 0
  spline S1106 degree 3 poles (58.909, 6.7777) (64.4119, 6.7777) (68.1959, 3.0471) (68.1959, -2.3768) knots 0 0 0 0 1 1 1 1
  spline S1107 degree 3 poles (68.1959, -2.3768) (68.1959, 3.0471) (64.4119, 6.7777) (58.909, 6.7777) knots -1 -1 -1 -1 0 0 0 0
  line L258 (-119.6048, 4.132) -> (-122.9922, -1.0805)
  line L259 (-122.9922, -1.0805) -> (-119.6048, 4.132)
  spline S1108 degree 3 poles (150.48, -10.3938) (150.48, -9.9969) (151.9352, -10.0763) (151.9352, -8.9386) knots 0 0 0 0 1 1 1 1
  spline S1109 degree 3 poles (151.9352, -8.9386) (151.9352, -10.0763) (150.48, -9.9969) (150.48, -10.3938) knots -1 -1 -1 -1 0 0 0 0
  spline S1110 degree 3 poles (-105.5281, 6.4337) (-104.7619, 6.4337) (-104.0221, 6.46) (-103.0944, 6.5129) knots 0 0 0 0 1 1 1 1
  spline S1111 degree 3 poles (-103.0944, 6.5129) (-104.0221, 6.46) (-104.7619, 6.4337) (-105.5281, 6.4337) knots -1 -1 -1 -1 0 0 0 0
  spline S1112 degree 3 poles (87.2182, 5.64) (87.2182, 5.2166) (85.9217, 5.296) (85.9217, 4.1583) knots 0 0 0 0 1 1 1 1
  spline S1113 degree 3 poles (85.9217, 4.1583) (85.9217, 5.296) (87.2182, 5.2166) (87.2182, 5.64) knots -1 -1 -1 -1 0 0 0 0
  spline S1114 degree 3 poles (69.888, -11.2669) (69.6763, -11.2934) (69.4117, -10.7113) (69.4117, -10.3938) knots 0 0 0 0 1 1 1 1
  spline S1115 degree 3 poles (69.4117, -10.3938) (69.4117, -10.7113) (69.6763, -11.2934) (69.888, -11.2669) knots -1 -1 -1 -1 0 0 0 0
  spline S1116 degree 3 poles (258.4795, 6.5131) (258.6912, 6.5131) (258.9558, 5.9575) (258.9558, 5.64) knots 0 0 0 0 1 1 1 1
  spline S1117 degree 3 poles (258.9558, 5.64) (258.9558, 5.9575) (258.6912, 6.5131) (258.4795, 6.5131) knots -1 -1 -1 -1 0 0 0 0
  spline S1118 degree 3 poles (-83.4111, -11.267) (-84.4664, -11.214) (-85.8448, -11.1903) (-87.2194, -11.1903) knots 0 0 0 0 1 1 1 1
  spline S1119 degree 3 poles (-87.2194, -11.1903) (-85.8448, -11.1903) (-84.4664, -11.214) (-83.4111, -11.267) knots -1 -1 -1 -1 0 0 0 0
  spline S1120 degree 3 poles (254.9606, -11.214) (253.1082, -11.214) (252.0234, -11.2934) (249.245, -11.2934) knots 0 0 0 0 1 1 1 1
  spline S1121 degree 3 poles (249.245, -11.2934) (252.0234, -11.2934) (253.1082, -11.214) (254.9606, -11.214) knots -1 -1 -1 -1 0 0 0 0
  spline S1122 degree 3 poles (70.7082, 2.0681) (70.7082, 3.7614) (70.5494, 4.8462) (70.2584, 5.64) knots 0 0 0 0 1 1 1 1
  spline S1123 degree 3 poles (70.2584, 5.64) (70.5494, 4.8462) (70.7082, 3.7614) (70.7082, 2.0681) knots -1 -1 -1 -1 0 0 0 0
  spline S1124 degree 3 poles (252.1822, -8.8328) (252.1822, -9.4942) (251.7853, -9.4413) (250.4624, -9.4413) knots -1 -1 -1 -1 0 0 0 0
  spline S1125 degree 3 poles (252.1822, -8.8328) (252.1822, -9.4942) (251.7853, -9.4413) (250.4624, -9.4413) knots -1 -1 -1 -1 0 0 0 0
  line L260 (-99.0459, -5.0229) -> (-103.0944, 6.5129)
  line L261 (-103.0944, 6.5129) -> (-99.0459, -5.0229)
  line L262 (70.7082, -8.9121) -> (70.7082, 2.0681)
  spline S1126 degree 3 poles (70.7082, 2.0681) (70.7082, 3.7614) (70.5494, 4.8462) (70.2584, 5.64) knots 0 0 0 0 1 1 1 1
  spline S1127 degree 3 poles (70.2584, 5.64) (70.1525, 5.931) (70.5494, 6.5395) (70.7611, 6.5131) knots 0 0 0 0 1 1 1 1
  spline S1128 degree 3 poles (70.7611, 6.5131) (72.6396, 6.3543) (74.0419, 6.5131) (74.915, 6.5131) knots 0 0 0 0 1 1 1 1
  spline S1129 degree 3 poles (74.915, 6.5131) (75.8675, 6.5131) (76.0263, 6.3014) (76.2909, 5.9045) knots 0 0 0 0 1 1 1 1
  line L263 (76.2909, 5.9045) -> (83.9373, -6.2928)
  line L264 (83.9373, -6.2928) -> (83.9373, 4.1583)
  spline S1130 degree 3 poles (83.9373, 4.1583) (83.9373, 5.296) (82.3498, 5.2166) (82.3498, 5.6135) knots 0 0 0 0 1 1 1 1
  spline S1131 degree 3 poles (82.3498, 5.6135) (82.3498, 5.931) (82.6409, 6.5395) (82.8525, 6.5131) knots 0 0 0 0 1 1 1 1
  spline S1132 degree 3 poles (82.8525, 6.5131) (83.2494, 6.4602) (84.0167, 6.4337) (84.784, 6.4337) knots 0 0 0 0 1 1 1 1
  spline S1133 degree 3 poles (84.784, 6.4337) (85.5513, 6.4337) (86.3186, 6.4602) (86.7419, 6.5131) knots 0 0 0 0 1 1 1 1
  spline S1134 degree 3 poles (86.7419, 6.5131) (86.9536, 6.5395) (87.2182, 5.9575) (87.2182, 5.64) knots 0 0 0 0 1 1 1 1
  spline S1135 degree 3 poles (87.2182, 5.64) (87.2182, 5.2166) (85.9217, 5.296) (85.9217, 4.1583) knots 0 0 0 0 1 1 1 1
  line L265 (85.9217, 4.1583) -> (85.9217, -8.9121)
  spline S1136 degree 3 poles (85.9217, -8.9121) (85.9217, -10.0498) (87.2182, -9.9705) (87.2182, -10.3673) knots 0 0 0 0 1 1 1 1
  spline S1137 degree 3 poles (87.2182, -10.3673) (87.2182, -10.6848) (86.9536, -11.3225) (86.7419, -11.2934) knots 0 0 0 0 1 1 1 1